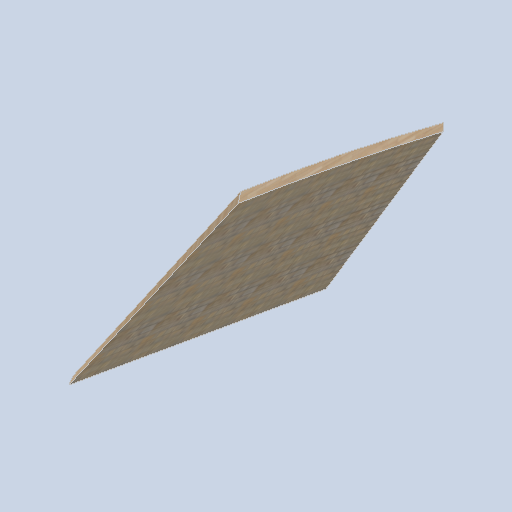
# Autodesk Inventor part: side_curve_panel_01
Saved by Autodesk Inventor 2024.2 (Build 282272000, 272)
## iProperties
Created: 2024-05-24
Part Number: side_curve_panel_01
Material: Wood (Maple)
Document SubType Name: Modeling
Designer: LOSTER_1
Density: 0.67 g/cm^3
Appearance: Natural Maple - Glossy Dark Tint
Author: LOSTER_1
Autodesk Inventor part; units mm, degrees
ref_plane "XZ Plane" through (0, 0, 0) normal (0, 1, 0) x (-1, 0, 0)
ref_plane "XY Plane" through (0, 0, 0) normal (0, 0, 1) x (1, 0, 0)
sketch "Sketch6" plane through (0, 0, 0) normal (1, 0, 0) x (0, 1, 0)
  arc A0 (55013.8042, -11170.4355) -> (55882.0451, -6246.3967) centre (-62703.3569, 12124.8427) ccw
  line L0 (55269.1589, -11215.4614) -> (56020.6222, -6953.7015)
  ellipse E0 centre (61810.8415, 1937.6455) end of major axis (51810.8415, 1937.9134) minor radius 9999.9998 (55920.4272, -6143.3827) -> (59138.8161, -7698.7583) ccw
  ellipse E1 centre (19401.1634, -2340.9962) end of major axis (39157.8615, -37121.3481) minor radius 39999.9568 (58289.9989, -11703.508) -> (59050.2828, -7627.3123) ccw construction
  ellipse E2 centre (19867.5037, -1667.5901) end of major axis (39624.2019, -36447.942) minor radius 39999.9568 (58483.7784, -12097.4311) -> (59393.074, -7809.8351) ccw
  line L1 (58220.5399, -12097.431) -> (58289.9989, -11703.508)
  line L2 (58483.7784, -12097.4311) -> (58220.5399, -12097.431)
  ellipse E3 centre (58713.4362, -7053.1537) end of major axis (59513.4362, -7053.1752) minor radius 800 (59125.2014, -7739.0469) -> (59401.1843, -7461.8131) ccw construction
  line L3 (59149.1724, -7692.8755) -> (59138.8161, -7698.7583) construction
  arc A1 (59124.9291, -7742.9966) -> (59375.6359, -7855.0237) centre (62717.5559, -39.5537) ccw construction
  ellipse E4 centre (59396.1726, -7809.0868) end of major axis (59346.1726, -7809.0854) minor radius 50 (59376.5228, -7855.0638) -> (59423.5807, -7850.9053) ccw construction
  point P0 (0, 0)
  constraints: 8 end point, 4 point on circle, 2 centre point, 20 other
ref_plane "Work Plane4" through (1791, 0, 0) normal (1, 0, 0) x (0, 1, 0)
ref_plane "Work Plane3" through (0, 0, 0) normal (1, 0, 0) x (0, 1, 0)
sketch "Sketch7" plane through (1791, 0, 0) normal (1, 0, 0) x (0, 1, 0)
  arc A0 (59221.5375, -7721.3143) -> (59399.6586, -7767.3118) centre (61810.8415, 1937.6455) ccw
  arc A1 (58588.0224, -11703.508) -> (59399.6586, -7767.3118) centre (19867.4824, -1667.6294) ccw
  line L0 (58439.0107, -11703.508) -> (58588.0224, -11703.508)
  arc A2 (58439.0107, -11703.508) -> (59221.5375, -7721.3143) centre (9808.9754, -79.4095) ccw
  point P0 (0, 0)
  point P1 (58289.9989, -11703.508)
  point P2 (59044.2926, -7672.0479)
  point P3 (58289.9989, -11703.508)
  dimension "d17" = 50000
  constraints: 6 point on circle, 3 centre point, 2 coincident, 2 end point, 1 horizontal
  measures "d17" radius of A2
sketch "Sketch8" plane through (0, 0, 0) normal (1, 0, 0) x (0, 1, 0)
  line L0 (55269.1589, -11215.4614) -> (56020.6222, -6953.7015) projected
  line L1 (55269.1589, -11215.4614) -> (56020.6222, -6953.7015)
  line L2 (56020.6222, -6953.7015) -> (56136.4974, -6296.5403)
  arc A0 (56017.7557, -6213.4375) -> (56136.4974, -6296.5403) centre (61810.8415, 1937.6455) ccw
  line L3 (55269.1589, -11215.4614) -> (55137.022, -11215.4614)
  line L4 (55137.022, -11215.4614) -> (56017.7557, -6213.4375)
  point P0 (0, 0)
  point P1 (55013.8042, -11170.4355)
  point P2 (55882.0451, -6246.3967)
  point P3 (58220.5399, -12097.431)
  point P4 (54826.5604, -12097.431)
  constraints: 8 end point, 2 point on circle, 1 centre point, 1 coincident, 1 collinear, 1 horizontal
loft "Loft3" add profiles "Sketch8", "Sketch7"
body "Solid3"
